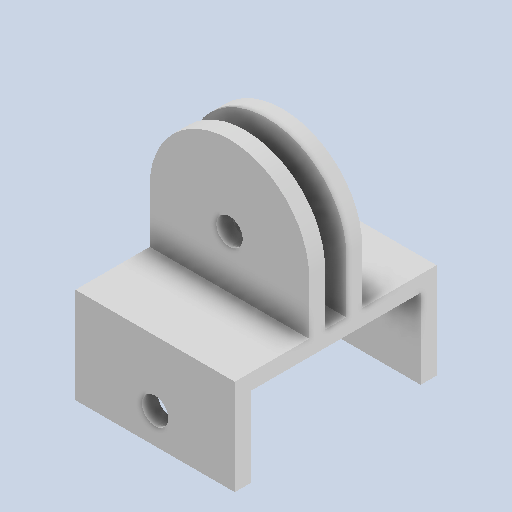
# Autodesk Inventor part: Sujetador_Carril
Saved by Autodesk Inventor 2022 (Build 260153000, 153)
## iProperties
Created: 2022-01-30
Part Number: Sujetador_Carril
Material: Generic
Document SubType Name: Modeling
Designer: katha
Density: 1 g/cm^3
Appearance: Default
Author: katha
Autodesk Inventor part; units mm, degrees
ref_plane "YZ Plane" through (0, 0, 0) normal (1, 0, 0) x (0, 1, 0)
ref_plane "XZ Plane" through (0, 0, 0) normal (0, 1, 0) x (-1, 0, 0)
ref_plane "XY Plane" through (0, 0, 0) normal (0, 0, 1) x (1, 0, 0)
sketch "Sketch2" plane through (0, 0, 0) normal (1, 0, 0) x (0, 1, 0)
  line L0 (0, -12.532) -> (0, 12.468) projected
  line L1 (0, 12.468) -> (3, 12.468) projected
  line L2 (3, -12.532) -> (3, 12.468) projected
  line L3 (0, -12.532) -> (3, -12.532) projected
  line L4 (-17, -12.532) -> (3, -12.532) projected
  line L5 (3, -12.532) -> (3, -15.532) projected
  line L6 (-17, -15.532) -> (3, -15.532) projected
  line L7 (-17, -12.532) -> (-17, -15.532) projected
  line L8 (3.5, -13.032) -> (3.5, -0.032)
  line L9 (-11.5, -16.032) -> (3.5, -16.032)
  line L10 (3.5, -13.032) -> (3.5, -16.032)
  line L11 (-11.5, -19.032) -> (6.5, -19.032)
  line L12 (3.5, -0.032) -> (6.5, -0.032) construction
  line L13 (-11.5, -16.032) -> (-11.5, -19.032)
  line L14 (6.5, -2.032) -> (31.5, -2.032)
  line L15 (31.5, -2.032) -> (31.5, -5.032)
  line L16 (31.5, -5.032) -> (6.5, -5.032)
  line L17 (3.5, 12.968) -> (3.5, -0.032)
  line L18 (-11.5, 15.968) -> (3.5, 15.968)
  line L19 (3.5, 12.968) -> (3.5, 15.968)
  line L20 (-11.5, 18.968) -> (6.5, 18.968)
  line L21 (-11.5, 15.968) -> (-11.5, 18.968)
  line L22 (6.5, 1.968) -> (31.5, 1.968)
  line L23 (31.5, 1.968) -> (31.5, 4.968)
  line L24 (31.5, 4.968) -> (6.5, 4.968)
  line L25 (3, 12.468) -> (-17, 12.468) projected
  line L26 (-17, 12.468) -> (-17, 15.468) projected
  line L27 (3, 15.468) -> (-17, 15.468) projected
  line L28 (3, 12.468) -> (3, 15.468) projected
  line L29 (6.5, 18.968) -> (6.5, 4.968)
  line L30 (6.5, 1.968) -> (6.5, -0.032)
  line L31 (6.5, -19.032) -> (6.5, -5.032)
  line L32 (6.5, -2.032) -> (6.5, -0.032)
  point P0 (0, 0)
  dimension "d0" = 0.5
  dimension "d1" = 0.5
  dimension "d3" = 15
  dimension "d4" = 3
  dimension "d5" = 19
  dimension "d7" = 25
  dimension "d8" = 2
  dimension "d9" = 3
  dimension "d11" = 3.5
  constraints: 42 end point, 9 symmetric about line, 4 perpendicular, 3 vertical, 1 collinear, 1 horizontal
  measures "d0" distance between parallel lines of L2 L8
  measures "d1" distance between parallel lines of L6 L9
  measures "d3" distance between parallel lines of L13 L10
  measures "d4" distance between parallel lines of L11 L9
  measures "d5" distance between parallel lines of L11 L12
  measures "d7" distance of L14.start L14.end
  measures "d8" distance between parallel lines of L14 L12
  measures "d9" distance of L14.end L15.end
  measures "d11" distance between parallel lines of L31 L2
extrude "Extrusion1" add sketch "Sketch2" along normal blind 15 and the other way blind 15 contours L8 L17 L19 L18 L21 L20 L29 L24 L23 L22 L30 L32 L14 L15 L16 L31 L11 L13 L9 L10
fillet "Fillet1" radius 15 4 edges at (-15, 31.5, -3.532) (-15, 31.5, 3.468) (15, 31.5, -3.532) (15, 31.5, 3.468)
sketch "Sketch3" plane through (15, 6.5, -19.032) normal (0, 0, -1) x (-1, 0, 0)
  line L0 (-110, -6.5) -> (140, -6.5) projected
  line L1 (0, -18) -> (30, -18) projected
  line L2 (0, -18) -> (0, 0) projected
  line L3 (30, 0) -> (30, -18) projected
  point P0 (15, -6.5)
  point P1 (15, -12.25)
  dimension "d17" = 5.75
  dimension "d18" = 15
  measures "d17" distance from line of point (15, -12.25) L1
  measures "d18" distance from line of L3 point (15, -12.25)
hole "Hole1" at (0, -5.75, -19.032) direction (0, 0, 1) diameter 5 depth 300 tip angle 118
sketch "Sketch4" plane through (15, 6.5, -5.032) normal (0, 0, -1) x (-1, 0, 0)
  arc A0 (30, 10) -> (0, 10) centre (15, 10) ccw projected
  point P0 (15, -6.5)
  constraints: 1 coincident
hole "Hole2" at (0, 16.5, -5.032) direction (0, 0, 1) diameter 5 depth 300 tip angle 118
body "Solid1"
